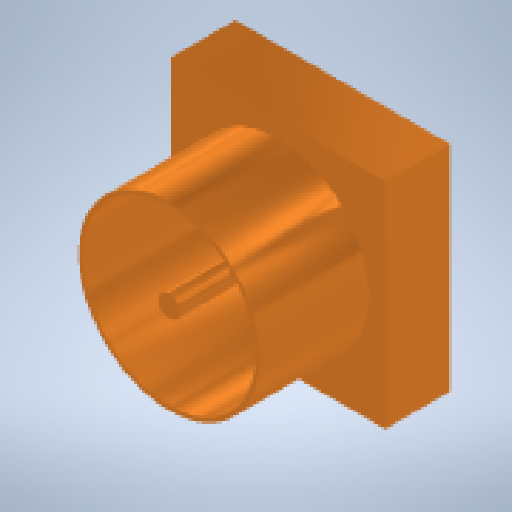
# Autodesk Inventor part: Connector
Saved by Autodesk Inventor 2023.1 (Build 271208000, 208)
## iProperties
Company: Aalto University / OtaNano
Created: 2023-05-15
Part Number: Connector
Material: Gold
Document SubType Name: Modeling
Designer: Joel Salminen
Mass: 0.672691 g
Surface Area: 1.54884 cm^2
Volume: 0.0348544 cm^3
Density: 19.3 g/cm^3
Appearance: Metal 1600F Hot
Author: Joel Salminen
Autodesk Inventor part; units mm, degrees
ref_plane "YZ Plane" through (0, 0, 0) normal (1, 0, 0) x (0, 1, 0)
ref_plane "XZ Plane" through (0, 0, 0) normal (0, 1, 0) x (-1, 0, 0)
ref_plane "XY Plane" through (0, 0, 0) normal (0, 0, 1) x (1, 0, 0)
sketch "Sketch1" plane through (0, 0, 0) normal (0, 0, 1) x (1, 0, 0)
  line L0 (2.485, 2.485) -> (-2.485, 2.485)
  line L1 (-2.485, 2.485) -> (-2.485, -2.485)
  line L2 (-2.485, -2.485) -> (2.485, -2.485)
  line L3 (2.485, -2.485) -> (2.485, 2.485)
  line L4 (2.485, 2.485) -> (-2.485, -2.485) construction
  line L5 (-2.485, 2.485) -> (2.485, -2.485) construction
  point P0 (0, 0)
  dimension "d0" = 4.97
  constraints: 12 end point, 2 midpoint, 2 parallel, 2 perpendicular, 1 horizontal
  measures "d0" distance of L2.end L1.end
extrude "Extrusion1" add sketch "Sketch1" along normal blind 1.5
sketch "Sketch2" plane through (0, 0, 1.5) normal (0, 0, 1) x (1, 0, 0)
  circle A0 centre (0, 0) radius 2.1
  dimension "d3" = 4.2
  constraints: 1 centre point, 1 coincident
  measures "d3" diameter of A0
extrude "Extrusion2" add sketch "Sketch2" along normal blind 2.52
sketch "Sketch3" plane through (0, 0, 4.02) normal (0, 0, 1) x (1, 0, 0)
  circle A0 centre (0, 0) radius 2.1 projected
  circle A1 centre (0, 0) radius 0.25
  circle A2 centre (0, 0) radius 2
  dimension "d6" = 0.5
  dimension "d7" = 4
  constraints: 2 centre point, 2 coincident
  measures "d6" diameter of A1
  measures "d7" diameter of A2
extrude "Extrusion3" cut sketch "Sketch3" against normal blind 3 contours A2
body "Solid1"
